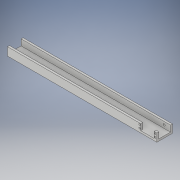
# Autodesk Inventor part: ArmProto1.2
Saved by Autodesk Inventor 2017 (Build 210142000, 142)
## iProperties
Created: 2017-09-30
Part Number: ArmProto1.2
Material: Generic
Document SubType Name: Modeling
Designer: User
Density: 1 g/cm^3
Appearance: Default
Author: User
Autodesk Inventor part; units mm, degrees
ref_plane "YZ Plane" through (0, 0, 0) normal (1, 0, 0) x (0, 1, 0)
ref_plane "XZ Plane" through (0, 0, 0) normal (0, 1, 0) x (-1, 0, 0)
ref_plane "XY Plane" through (0, 0, 0) normal (0, 0, 1) x (1, 0, 0)
sketch "Sketch1" plane through (0, 0, 0) normal (1, 0, 0) x (0, 1, 0)
  line L0 (0, 0) -> (25.4, 0)
  line L1 (25.4, 0) -> (25.4, -49.149)
  line L2 (25.4, -49.149) -> (0, -49.149)
  line L3 (0, -49.149) -> (0, 0)
  line L4 (25.4, -6.35) -> (6.35, -6.35)
  line L5 (6.35, -6.35) -> (6.35, -42.799)
  line L6 (6.35, -42.799) -> (25.4, -42.799)
  line L7 (25.4, -42.799) -> (25.4, -6.35)
  dimension "d0" = 25.4
  dimension "d1" = 49.149
  dimension "d2" = 19.05
  dimension "d3" = 36.449
  dimension "d4" = 6.35
  constraints: 16 end point, 4 parallel, 2 horizontal, 2 perpendicular, 1 point on line
  measures "d0" distance of L1.end L2.end
  measures "d1" distance of L0.end L1.end
  measures "d2" distance of L5.end L6.end
  measures "d3" distance of L4.end L5.end
  measures "d4" distance between parallel lines of L0 L4
extrude "Extrusion1" add sketch "Sketch1" along normal blind 469.9 contours L0 L1 L4 L5 L6 L2 L3
sketch "Sketch2" plane through (0, 0, 0) normal (0, 0, 1) x (1, 0, 0)
  line L0 (0, 25.4) -> (0, 0) projected
  line L1 (0, 0) -> (469.9, 0) projected
  line L2 (469.9, 25.4) -> (469.9, 0) projected
  line L3 (0, 25.4) -> (469.9, 25.4) projected
  line L4 (461.01, 25.4) -> (419.1, 25.4)
  line L5 (419.1, 25.4) -> (419.1, 6.35)
  line L6 (419.1, 6.35) -> (461.01, 6.35)
  line L7 (461.01, 6.35) -> (461.01, 25.4)
  circle A0 centre (464.8962, 21.2344) radius 2.413
  circle A1 centre (464.8962, 11.2268) radius 2.413
  circle A2 centre (415.6202, 21.2344) radius 2.413
  circle A3 centre (415.6202, 11.2268) radius 2.413
  dimension "d7" = 8.89
  dimension "d8" = 25.4
  dimension "d9" = 19.05
  dimension "d10" = 50.8
  dimension "d11" = 4.826
  dimension "d12" = 4.826
  dimension "d13" = 4.1656
  dimension "d14" = 10.0076
  dimension "d15" = 4.826
  dimension "d16" = 4.826
  dimension "d17" = 54.2798
  dimension "d18" = 54.2798
  dimension "d26" = 5.0038
  dimension "d27" = 5.0038
  constraints: 8 end point, 4 centre point, 2 parallel, 1 horizontal, 1 perpendicular, 1 point on line
  measures "d7" distance between parallel lines of L2 L7
  measures "d8" distance of L2.start L1.end
  measures "d9" distance of L6.end L4.start
  measures "d10" distance between parallel lines of L2 L5
  measures "d11" diameter of A0
  measures "d12" diameter of A1
  measures "d13" distance from line of A0.centre L3
  measures "d14" distance of A1.centre A0.centre
  measures "d15" diameter of A2
  measures "d16" diameter of A3
  measures "d17" distance from line of L2 A2.centre
  measures "d18" distance from line of L2 A3.centre
  measures "d26" distance from line of L2 A0.centre
  measures "d27" distance from line of L2 A1.centre
extrude "Extrusion2" cut sketch "Sketch2" against normal blind 12.7 contours L3 L7 L6 L5 | A0 | A1 | A2 | A3
sketch "Sketch3" plane through (0, 0, -49.149) normal (0, 0, -1) x (-1, 0, 0)
  line L0 (0, 0) -> (0, 25.4) projected
  line L1 (0, 25.4) -> (-469.9, 25.4) projected
  line L2 (-469.9, 0) -> (-469.9, 25.4) projected
  line L3 (0, 0) -> (-469.9, 0) projected
  circle A0 centre (-450.1896, 16.2306) radius 3.175
  point P0 (0, 0)
  dimension "d21" = 6.35
  dimension "d22" = 19.7104
  dimension "d23" = 9.1694
  constraints: 1 centre point
  measures "d21" diameter of A0
  measures "d22" distance from line of L2 A0.centre
  measures "d23" distance from line of L1 A0.centre
extrude "Extrusion3" cut sketch "Sketch3" against normal blind 12.7 contours A0
equation "\"d12\" = d11"
equation "\"d15\" = d11"
equation "\"d16\" = d11"
equation "\"d18\" = d17"
equation "\"d27\" = d26"
body "Solid1"
